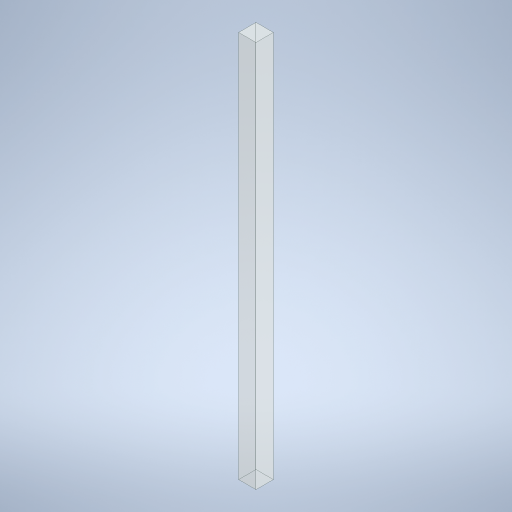
# Autodesk Inventor part: Chimney
Saved by Autodesk Inventor 2024 (Build 280153000, 153)
## iProperties
Created: 2023-05-18
Part Number: Chimney
Material: Concrete
Document SubType Name: Modeling
Designer: Tom
Density: 2.40731 g/cm^3
Appearance: Clear
Author: Tom
Autodesk Inventor part; units mm, degrees
ref_plane "YZ Plane" through (0, 0, 0) normal (1, 0, 0) x (0, 1, 0)
ref_plane "XZ Plane" through (0, 0, 0) normal (0, 1, 0) x (-1, 0, 0)
ref_plane "XY Plane" through (0, 0, 0) normal (0, 0, 1) x (1, 0, 0)
sketch "Sketch1" plane through (0, 0, 0) normal (0, 1, 0) x (-1, 0, 0)
  line L0 (0, 0) -> (406.4, 0)
  line L1 (406.4, 0) -> (406.4, -406.4)
  line L2 (406.4, -406.4) -> (0, -406.4)
  line L3 (0, -406.4) -> (0, 0)
  dimension "d1" = 406.4
  dimension "d2" = 406.4
  constraints: 8 end point, 2 parallel, 1 horizontal, 1 perpendicular
  measures "d1" distance of L0.start L0.end
  measures "d2" distance of L2.end L0.start
extrude "Extrusion1" add sketch "Sketch1" along normal blind 9048.75
body "Solid1"
